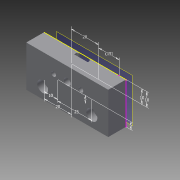
# Autodesk Inventor part: detalKKoretke
Saved by Autodesk Inventor 2015 (Build 190159000, 159)
## iProperties
Created: 2016-04-08
Part Number: detalKKoretke
Material: Generic
Document SubType Name: Modeling
Designer: Andreas
Density: 1 g/cm^3
Appearance: Default
Author: Andreas
Autodesk Inventor part; units mm, degrees
ref_plane "YZ Plane" through (0, 0, 0) normal (1, 0, 0) x (0, 1, 0)
ref_plane "XZ Plane" through (0, 0, 0) normal (0, 1, 0) x (-1, 0, 0)
ref_plane "XY Plane" through (0, 0, 0) normal (0, 0, 1) x (1, 0, 0)
sketch "Sketch1" plane through (0, 0, 0) normal (0, 1, 0) x (-1, 0, 0)
  line L0 (0, 0) -> (60, 0)
  line L1 (60, 0) -> (60, -30)
  line L2 (60, -30) -> (0, -30)
  line L3 (0, -30) -> (0, 0)
  dimension "d0" = 60
  dimension "d1" = 30
  dimension "d2" = 60
  constraints: 8 end point, 2 perpendicular, 1 horizontal
  measures "d0" distance of L0.start L0.end
  measures "d1" distance of L0.end L1.end
  measures "d2" distance of L1.end L2.end
extrude "Extrusion1" add sketch "Sketch1" against normal blind 5 and the other way blind 10
sketch "Sketch2" plane through (0, 10, 0) normal (0, 1, 0) x (1, 0, 0)
  line L0 (-60, 30) -> (-60, 0) projected
  line L1 (0, 0) -> (0, 30) projected
  line L2 (0, 30) -> (-60, 30) projected
  line L3 (-60, 0) -> (0, 0) projected
  line L4 (-5, 0) -> (-5, 30) projected
  point P0 (-40, 10)
  point P1 (-20, 10)
  dimension "d44" = 10
  dimension "d45" = 20
  dimension "d46" = 20
  dimension "d47" = 10
  dimension "d67" = 15
  measures "d44" distance from line of L3 point (-40, 10)
  measures "d45" distance from line of L0 point (-40, 10)
  measures "d46" distance of point (-40, 10) point (-20, 10)
  measures "d47" distance from line of L3 point (-20, 10)
  measures "d67" distance from line of L4 point (-20, 10)
sketch "Sketch3" plane through (0, 10, 0) normal (0, 1, 0) x (1, 0, 0)
  line L0 (0, 30) -> (-60, 30) projected
  line L1 (-60, 0) -> (-60, 30) projected
  point P0 (0, 0)
  point P1 (-50, 25)
  point P2 (-5, 30)
  point P3 (-25, 25)
  dimension "d56" = 5
  dimension "d57" = 10
  dimension "d58" = 25
  dimension "d59" = 5
  measures "d56" distance from line of L0 point (-50, 25)
  measures "d57" distance from line of L1 point (-50, 25)
  measures "d58" distance of point (-50, 25) point (-25, 25)
  measures "d59" distance from line of L0 point (-25, 25)
sketch "Sketch16" plane through (-60, -5, 0) normal (0, 0, 1) x (1, 0, 0)
  line L0 (60, 15) -> (0, 15) projected
  line L1 (24.5, 15) -> (25.5, 15)
  line L2 (25.5, 15) -> (25.5, 14.25)
  line L3 (25.5, 14.25) -> (24.5, 14.25)
  line L4 (24.5, 14.25) -> (24.5, 12)
  line L5 (24.5, 12) -> (35.5, 12)
  line L6 (35.5, 12) -> (35.5, 14.25)
  line L7 (35.5, 14.25) -> (34.5, 14.25)
  line L8 (34.5, 14.25) -> (34.5, 15)
  line L9 (35.5, 15) -> (24.5, 15)
  line L10 (60, 0) -> (0, 0) projected
  line L11 (0, 15) -> (60, 15) projected
  point P0 (60, 5)
  point P1 (30, 15)
  point P2 (30, 0)
  point P3 (30, 15)
  point P4 (30, 0)
  point P5 (30, 15)
  point P6 (30, 0)
  dimension "d90" = 1
  dimension "d91" = 0.75
  dimension "d92" = 2.25
  dimension "d93" = 11
  dimension "d94" = 1
  dimension "d138" = 1
  constraints: 18 end point, 7 point on line, 6 midpoint, 6 perpendicular, 3 vertical alignment, 1 collinear
  measures "d90" distance of L1.start L1.end
  measures "d91" distance of L1.end L2.end
  measures "d92" distance of L3.end L4.end
  measures "d93" distance of L4.end L5.end
  measures "d94" distance of L6.end L7.end
  measures "d138" distance between parallel lines of L4 L2
extrude "Extrusion6" cut sketch "Sketch16" against normal up to next
sketch "Sketch17" plane through (-35.5, 7, 0) normal (0, 1, 0) x (1, 0, 0)
  circle A0 centre (5.5, 10) radius 2.5
  line L0 (0, 30) -> (11, 30) projected
  point P0 (35.5, 0)
  point P1 (5.5, 30)
  dimension "d97" = 5
  constraints: 1 centre point, 1 midpoint, 1 vertical alignment
  measures "d97" diameter of A0
extrude "Extrusion7" cut sketch "Sketch17" against normal up to next
ref_plane "Work Plane2" through (0, 13.5, 0) normal (0, 1, 0) x (1, 0, 0)
sketch "Sketch21" plane through (0, -5, 0) normal (0, -1, 0) x (1, 0, 0)
  circle A0 centre (-12, -22) radius 4
  circle A1 centre (-48, -22) radius 4
  point P0 (0, 0)
  dimension "d125" = 8
  dimension "d131" = 8
  constraints: 2 centre point
  measures "d125" diameter of A0
  measures "d131" diameter of A1
extrude "Extrusion13" cut sketch "Sketch21" against normal blind 10
sketch "Sketch23" plane through (-12, 5, -22) normal (0, -1, 0) x (1, 0, 0)
  circle A0 centre (0, 0) radius 1.5
  circle A1 centre (-36, 0) radius 1.5
  point P0 (12, 22)
  dimension "d134" = 3
  dimension "d135" = 3
  constraints: 2 centre point
  measures "d134" diameter of A0
  measures "d135" diameter of A1
extrude "Extrusion14" cut sketch "Sketch23" against normal up to next
sketch "Sketch24" plane through (0, 10, 0) normal (0, 1, 0) x (1, 0, 0)
  circle A0 centre (-40, 10) radius 1.5
  circle A1 centre (-20, 10) radius 1.5
  point P0 (0, 0)
  dimension "d143" = 3
  dimension "d144" = 3
  constraints: 2 centre point
  measures "d143" diameter of A0
  measures "d144" diameter of A1
extrude "Extrusion15" cut sketch "Sketch24" against normal up to next
sketch "Sketch11" plane through (0, 10, 0) normal (0, 1, 0) x (1, 0, 0)
  point P0 (-20, 10)
  point P1 (-40, 10)
body "Solid1"
